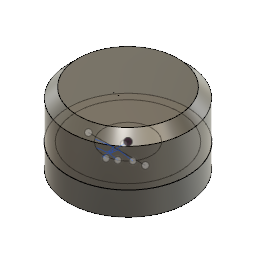
d-shaft-knob (Autodesk Fusion 360 design; units mm, degrees)
Autodesk Fusion 360 part; units mm, degrees
note: some values were not read from the file. Set by a fixed rule: which sketch regions a step uses.
sketch "Sketch1" plane through (0, 0, 0) normal (0, 1, 0) x (1, 0, 0)
  circle A0 centre (0, 0) radius 3
  circle A1 centre (0, 0) radius 6.5
  circle A2 centre (0, 0) radius 7.5
  line L0 (-3.5081, -1.5) -> (3.6969, -1.5)
  line L1 (-2.4042, -1.7943) -> (-0.3233, -1.5)
  line L2 (-0.1362, -2.4721) -> (-1.3744, -2.6666)
  line L3 (-0.1362, -2.4721) -> (-0.2747, -1.4931)
  line L4 (-0.0006, -0.4974) -> (-0.0006, -3.2095)
  line L5 (-0.0006, -3.2095) -> (0.4355, -3.2095)
  line L6 (2.403, -1.7943) -> (0.3221, -1.5)
  line L7 (0.135, -2.4721) -> (0.2735, -1.4931)
  line L8 (0.135, -2.4721) -> (1.3732, -2.6666)
  line L9 (0.3221, -1.5) -> (0.2735, -1.4931)
  line L10 (-0.3233, -1.5) -> (-0.2747, -1.4931)
  line L11 (1.3732, -2.6666) -> (1.3779, -2.6674)
  line L12 (2.403, -1.7943) -> (2.4082, -1.7951)
  dimension "d1" = 6
  dimension "d2" = 13
  dimension "d3" = 15
  dimension "d4" = 1.5
  dimension "d5" = 0.4361
  measures "d1" diameter of A0
  measures "d2" diameter of A1
  measures "d3" diameter of A2
  measures "d4" distance of A0.centre L0
  measures "d5" distance of L4.end L5.end
extrude "Extrude5" add sketch "Sketch1" along normal blind 1 contours A0 L0 L1 L2 L3 | A0 L0 L1 | A0 L0 L2 L3 L4 | A0 L0 L3 L7 L9 L10 | A0 L0 L4 L7 L8 | A0 L0 L6 L7 L8 | A0 L0 L6 | A1 | A2 makes body 1
extrude "Extrude2" add sketch "Sketch1" along normal blind 5 separate body contours A0 L0 L6 L7 L8 makes body 2
extrude "Extrude1" add sketch "Sketch1" along normal blind 5 separate body contours A0 L0 L1 L2 L3 makes body 3
extrude "Extrude3" add sketch "Sketch1" along normal blind 5 contours A1 bodies 2 3
extrude "Extrude4" add sketch "Sketch1" along normal blind -3 and the other way blind -5 separate body contours A2 makes body 4
move_body "Move1" bodies 1 to x (1, 0, 0) y (0, 1, 0) z (0, 0, 1) at (0, 5, 0)
combine "Combine1" operation add target body 4 tool bodies 1 2
chamfer "Chamfer1" distance 1.2 angle 45 1 edges at (-6.9925, 6, 2.7121) on bodies 4
named bodies: "knob"
